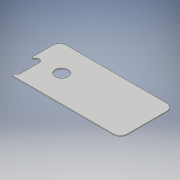
# Autodesk Inventor part: Google Pixel - Clear Case Cutout
Saved by Autodesk Inventor 2018 (Build 220112000, 112)
## iProperties
Created: 2017-10-04
Part Number: Google Pixel - Clear Case Cutout
Material: Generic
Document SubType Name: Modeling
Designer: xdlea
Density: 1 g/cm^3
Appearance: Default
Author: xdlea
Autodesk Inventor part; units mm, degrees
ref_plane "YZ Plane" through (0, 0, 0) normal (1, 0, 0) x (0, 1, 0)
ref_plane "XZ Plane" through (0, 0, 0) normal (0, 1, 0) x (-1, 0, 0)
ref_plane "XY Plane" through (0, 0, 0) normal (0, 0, 1) x (1, 0, 0)
sketch "Sketch1" plane through (0, 0, 0) normal (0, 1, 0) x (-1, 0, 0)
  line L0 (-75, 35) -> (-66, 35) construction
  line L1 (75, 35) -> (75, 26) construction
  line L2 (75, -35) -> (66, -35) construction
  line L3 (-75, -35) -> (-75, -26) construction
  line L4 (-75, 35) -> (75, -35) construction
  line L5 (75, 35) -> (-75, -35) construction
  arc A0 (75, 26) -> (66, 35) centre (66, 26) ccw construction
  arc A1 (66, -35) -> (75, -26) centre (66, -26) ccw
  arc A2 (-75, -26) -> (-66, -35) centre (-66, -26) ccw
  arc A3 (-66, 35) -> (-75, 26) centre (-66, 26) ccw
  line L6 (75, 26) -> (75, 0.5) construction
  line L7 (66, 35) -> (75, 35) construction
  line L8 (-66, 35) -> (66, 35)
  line L9 (-75, 26) -> (-75, 35) construction
  line L10 (-75, -26) -> (-75, 26)
  line L11 (-66, -35) -> (-75, -35) construction
  line L12 (66, -35) -> (-66, -35)
  line L13 (75, -26) -> (75, -35) construction
  circle A4 centre (37.25, 0) radius 8.25
  line L14 (64, 27.375) -> (64, 2.875)
  arc A5 (66.7085, 31.4202) -> (66, 35) centre (66, 33.14) ccw
  arc A6 (64, 2.875) -> (72.3603, 1.0699) centre (68.375, 2.875) ccw
  arc A7 (75, 0.5) -> (72.3603, 1.0699) centre (73.6186, 0.5) ccw
  line L15 (66, 35) -> (66, 35) construction
  line L16 (75, 0.5) -> (75, -26)
  arc A8 (66.7085, 31.4202) -> (64, 27.375) centre (68.375, 27.375) ccw
  point P0 (0, 0)
  point P1 (0, 0)
  dimension "d3" = 70
  dimension "d4" = 150
  dimension "d5" = 16.5
  dimension "d6" = 29.5
  dimension "d7" = 11
  dimension "d10" = 4.375
  dimension "d14" = 36.5
  dimension "d15" = 3.25
  dimension "d17" = 2.375
  dimension "d19" = 9
  dimension "d21" = 2.375
  constraints: 37 tangent, 34 end point, 24 parallel, 16 perpendicular, 16 point on circle, 9 centre point, 4 equal radius, 4 horizontal, 3 midpoint, 1 horizontal alignment, 1 point on line, 1 vertical
  measures "d3" distance of L3.start L0.start
  measures "d4" distance of L0.start L1.start
  measures "d5" diameter of A4
  measures "d6" distance edge to line of A4 L6
  measures "d7" distance between parallel lines of L14 L6
  measures "d10" radius of A6
  measures "d15" distance edge to line of A8 L8
  measures "d17" horizontal distance of A5.centre A8.centre
  measures "d19" horizontal distance of L13.start L2.end
  measures "d21" vertical distance of A7.centre A6.centre
extrude "Extrusion1" add sketch "Sketch1" along normal blind 1
body "Solid1"
